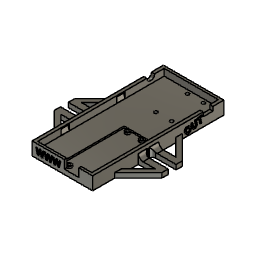
Attenuator case v8 (Autodesk Fusion 360 design; units mm, degrees)
Autodesk Fusion 360 part; units mm, degrees
note: some values were not read from the file. Set by a fixed rule: which sketch regions a step uses.
ref_plane "WorkPlane1" through (0, -11.43, -8.12) normal (0, 0, -1) x (0, -1, 0)
ref_plane "WorkPlane2" through (-25.8395, 48.6908, -2.3241) normal (-1, 0, 0) x (0, 0, 1)
ref_plane "WorkPlane3" through (-2.2175, 54.0502, -2.1844) normal (1, 0, 0) x (0, 1, 0)
sketch "Sketch2" plane through (-25.8395, 48.6908, -2.3241) normal (-1, 0, 0) x (0, 1, 0)
  line L0 (-7.62, -7.62) -> (10.16, -7.62)
  constraint horizontal L0
sketch "Sketch1" plane through (0, -11.43, -8.12) normal (0, 0, -1) x (1, 0, 0)
  line L0 (21.4045, -77.7992) -> (-25.8395, -77.7992)
  line L1 (-25.8395, -77.7992) -> (-25.8395, 28.04)
  line L2 (-25.8395, 28.04) -> (21.4045, 28.04)
  line L3 (21.4045, 28.04) -> (21.4045, -77.7992)
  line L4 (21.4045, -62.1782) -> (21.4045, -68.7822)
  line L5 (-25.8395, -52.5008) -> (-25.8395, -70.2808)
  line L6 (-0.4395, -75.2592) -> (-3.9955, -75.2592)
  line L7 (-10.5, 25.5) -> (10.5, 25.5)
  line L8 (-25.8395, -77.7992) -> (-26.6015, -77.7992)
  line L9 (-26.6015, -77.7992) -> (-26.6015, 28.04)
  line L10 (-26.6015, 28.04) -> (-25.8395, 28.04)
  line L11 (-25.8395, 28.04) -> (-25.8395, -77.7992)
  line L12 (21.4045, -77.7992) -> (22.1665, -77.7992)
  line L13 (22.1665, -77.7992) -> (22.1665, 28.04)
  line L14 (22.1665, 28.04) -> (21.4045, 28.04)
  line L15 (21.4045, 28.04) -> (21.4045, -77.7992)
  dimension "d10" = 2.54
  dimension "d11" = 2.54
  dimension "d12" = 0.762
  dimension "d13" = 0.762
  constraint horizontal L0
  constraint vertical L1
  constraint horizontal L2
  constraint vertical L3
  constraint collinear L3 L4
  constraint collinear L1 L5
  constraint horizontal L8
  constraint vertical L9
  constraint horizontal L10
  constraint vertical L11
  constraint collinear L2 L10
  constraint horizontal L12
  constraint vertical L13
  constraint horizontal L14
  constraint vertical L15
  constraint collinear L2 L14
  measures "d10" distance of L0 L6
  measures "d11" distance of L2 L7
  measures "d12" distance of L0.end L8.end
  measures "d13" distance of L0.start L12.end
extrude "Extrude2" add sketch "Sketch1" along normal blind 5.04
sketch "Sketch3" plane through (0, 0, -8.12) normal (0, 0, 1) x (-1, 0, 0)
  line L0 (-22.1665, -66.3692) -> (26.6015, -66.3692)
  line L1 (26.6015, -66.3692) -> (26.6015, 39.47)
  line L2 (26.6015, 39.47) -> (-22.1665, 39.47)
  line L3 (-22.1665, 39.47) -> (-22.1665, -66.3692)
  line L4 (26.6015, -66.3692) -> (-22.1665, -66.3692)
  line L5 (-22.1665, -66.3692) -> (-22.1665, 39.47)
  line L6 (-22.1665, 39.47) -> (26.6015, 39.47)
  line L7 (26.6015, 39.47) -> (26.6015, -66.3692)
  line L8 (25.3315, -64.4642) -> (-20.8965, -64.4642)
  line L9 (-20.8965, -64.4642) -> (-20.8965, 37.565)
  line L10 (-20.8965, 37.565) -> (25.3315, 37.565)
  line L11 (25.3315, 37.565) -> (25.3315, -64.4642)
  dimension "d16" = 1.905
  dimension "d17" = 1.905
  dimension "d18" = 1.27
  dimension "d19" = 1.27
  constraint horizontal L4
  constraint vertical L5
  constraint horizontal L6
  constraint vertical L7
  constraint coincident L2.end L3.start
  constraint coincident L0.end L1.start
  constraint horizontal L8
  constraint vertical L9
  constraint horizontal L10
  constraint vertical L11
  measures "d16" distance of L4 L8
  measures "d17" distance of L6 L10
  measures "d18" distance of L7 L11
  measures "d19" distance of L5 L9
extrude "Extrude3" add sketch "Sketch3" along normal blind 5.4356
sketch "Sketch4" plane through (22.1665, 0, 0) normal (1, 0, 0) x (0, 1, 0)
  line L0 (-39.47, -2.6844) -> (-39.47, -13.16)
  line L1 (-39.47, -13.16) -> (66.3692, -13.16)
  line L2 (66.3692, -13.16) -> (66.3692, -2.6844)
  line L3 (66.3692, -2.6844) -> (-39.47, -2.6844)
  circle A0 centre (53.6692, -2.6844) radius 3.175
  dimension "d22" = 6.35
  dimension "d23" = 12.7
  constraint coincident L3 A0.centre
  measures "d22" diameter of A0
  measures "d23" distance of L2 A0.centre
extrude "Extrude4" cut sketch "Sketch4" against normal up to surface (48.768 mm away) contours L3 A0 | L3 A0
sketch "Sketch5" plane through (22.1665, 0, 0) normal (1, 0, 0) x (0, 1, 0)
  arc A0 (50.4942, -2.6844) -> (56.8442, -2.6844) centre (53.6692, -2.6844) ccw
  line L0 (50.4942, -2.6844) -> (-39.47, -2.6844)
  line L1 (-39.47, -2.6844) -> (-39.47, -13.16)
  line L2 (-39.47, -13.16) -> (66.3692, -13.16)
  line L3 (66.3692, -13.16) -> (66.3692, -2.6844)
  line L4 (66.3692, -2.6844) -> (56.8442, -2.6844)
  line L5 (49.7322, -2.6844) -> (57.6062, -2.6844)
  line L6 (57.6062, -2.6844) -> (57.6062, -6.0198)
  line L7 (57.6062, -6.0198) -> (49.7322, -6.0198)
  line L8 (49.7322, -6.0198) -> (49.7322, -2.6844)
  line L9 (50.7482, 1.016) -> (57.3522, 1.016)
  line L10 (50.7482, 1.016) -> (50.7482, -5.3848)
  line L11 (57.3522, 1.016) -> (57.3522, -5.3848)
  line L12 (50.7482, -5.3848) -> (57.3522, -5.3848)
  dimension "d137" = 7.874
  dimension "d138" = 3.3354
  dimension "d139" = 8.763
  constraint horizontal L5
  constraint vertical L6
  constraint horizontal L7
  constraint vertical L8
  constraint collinear L4 L5
  measures "d137" distance of L6.end L7.end
  measures "d138" distance of L4 L7
  measures "d139" distance of L3 L6
extrude "Extrude5" cut sketch "Sketch5" against normal up to surface (1.27 mm away) contours A0 L0 L4 L5 L6 L7 L8 L10 L11 L12 | A0 L10 L12 | A0 L4 L5 L11 L12
sketch "Sketch10" plane through (0, -39.47, 0) normal (0, -1, 0) x (1, 0, 0)
  line L0 (22.1665, -2.6844) -> (-26.6015, -2.6844)
  line L1 (-26.6015, -2.6844) -> (-26.6015, -13.16)
  line L2 (-26.6015, -13.16) -> (22.1665, -13.16)
  line L3 (22.1665, -13.16) -> (22.1665, -2.6844)
  line L4 (-0.4634, -2.6844) -> (10.9837, -2.6844)
  line L5 (10.9837, -2.6844) -> (10.9837, -13.16)
  line L6 (10.9837, -13.16) -> (-0.4634, -13.16)
  line L7 (-0.4634, -13.16) -> (-0.4634, -2.6844)
  constraint horizontal L4
  constraint vertical L5
  constraint horizontal L6
  constraint vertical L7
  constraint coincident L2 L5.end
extrude "Extrude9" cut sketch "Sketch10" against normal up to surface (1.905 mm away) contours L0 L2 L4 L5 L6 L7
sketch "Sketch11" plane through (0, 0, -13.16) normal (0, 0, -1) x (1, 0, 0)
  line L0 (10.9837, 39.47) -> (10.9837, 37.565)
  line L1 (10.9837, 37.565) -> (-0.4634, 37.565)
  line L2 (-0.4634, 37.565) -> (-0.4634, 39.47)
  line L3 (-0.4634, 39.47) -> (-26.6015, 39.47)
  line L4 (-26.6015, 39.47) -> (-26.6015, -66.3692)
  line L5 (-26.6015, -66.3692) -> (22.1665, -66.3692)
  line L6 (22.1665, -66.3692) -> (22.1665, 39.47)
  line L7 (22.1665, 39.47) -> (10.9837, 39.47)
  line L8 (-26.6015, 2.64) -> (-45.6515, 2.64)
  line L9 (-45.6515, 2.64) -> (-45.6515, -13.87)
  line L10 (-45.6515, -13.87) -> (-26.6015, -13.87)
  line L11 (-26.6015, -13.87) -> (-26.6015, 2.64)
  line L12 (-45.6515, -8.79) -> (-26.6015, -8.79)
  line L13 (-26.6015, -8.79) -> (-26.6015, -2.44)
  line L14 (-26.6015, -2.44) -> (-45.6515, -2.44)
  line L15 (-45.6515, -2.44) -> (-45.6515, -8.79)
  line L16 (22.1665, 2.64) -> (41.2165, 2.64)
  line L17 (41.2165, 2.64) -> (41.2165, -13.87)
  line L18 (41.2165, -13.87) -> (22.1665, -13.87)
  line L19 (22.1665, -13.87) -> (22.1665, 2.64)
  line L20 (22.1665, -2.44) -> (41.2165, -2.44)
  line L21 (41.2165, -2.44) -> (41.2165, -8.79)
  line L22 (41.2165, -8.79) -> (22.1665, -8.79)
  line L23 (22.1665, -8.79) -> (22.1665, -2.44)
  line L24 (-45.6515, 2.64) -> (-26.6015, 21.69)
  line L25 (-45.6515, 2.64) -> (-18.7108, 2.64) construction
  line L26 (-40.2634, 2.64) -> (-26.6015, 16.3018)
  line L27 (-45.6515, -13.87) -> (-26.6015, -32.92)
  line L28 (-45.6515, -13.87) -> (-18.7108, -13.87) construction
  line L29 (-40.2634, -13.87) -> (-26.6015, -27.5318)
  line L30 (41.2165, -13.87) -> (22.1665, -32.92)
  line L31 (41.2165, -13.87) -> (68.1572, -13.87) construction
  line L32 (35.8283, -13.87) -> (22.1665, -27.5318)
  line L33 (41.2165, 2.64) -> (22.1665, 21.69)
  line L34 (35.8283, 2.64) -> (22.1665, 16.3018)
  dimension "d46" = 16.51
  dimension "d47" = 6.35
  dimension "d48" = 36.83
  dimension "d49" = 19.05
  dimension "d107" = 45
  dimension "d108" = 3.81
  dimension "d109" = 45
  dimension "d110" = 3.81
  dimension "d111" = 135
  constraint horizontal L8
  constraint vertical L9
  constraint horizontal L10
  constraint vertical L11
  constraint coincident L4 L8.start
  constraint horizontal L12
  constraint vertical L13
  constraint horizontal L14
  constraint vertical L15
  constraint coincident L4 L13.end
  constraint coincident L9 L12.start
  constraint horizontal L16
  constraint vertical L17
  constraint horizontal L18
  constraint vertical L19
  constraint coincident L6 L16.start
  constraint horizontal L20
  constraint vertical L21
  constraint horizontal L22
  constraint vertical L23
  constraint coincident L17 L21.end
  constraint coincident L6 L20.start
  constraint collinear L8 L16
  constraint collinear L10 L18
  constraint collinear L12 L22
  constraint collinear L14 L20
  constraint midpoint L11 L13
  constraint equal L8 L16
  constraint horizontal L25
  constraint coincident L4 L24.end
  constraint coincident L25 L26.start
  constraint coincident L4 L26.end
  constraint parallel L24 L26
  constraint horizontal L28
  constraint coincident L4 L27.end
  constraint coincident L28 L29.start
  constraint coincident L4 L29.end
  constraint parallel L27 L29
  constraint horizontal L31
  constraint coincident L6 L30.end
  constraint coincident L18 L32.start
  constraint coincident L6 L32.end
  constraint parallel L30 L32
  constraint coincident L6 L33.end
  constraint perpendicular L32 L33
  constraint coincident L16 L34.start
  constraint coincident L6 L34.end
  constraint parallel L33 L34
  constraint equal L26 L34
  constraint equal L29 L32
  measures "d46" distance of L8.end L9.end
  measures "d47" distance of L12.start L14.end
  measures "d48" distance of L3.end L8.start
  measures "d49" distance of L8.start L8.end
  measures "d107" angle of L24 L25
  measures "d108" distance of L24 L26
  measures "d109" angle of L27 L28
  measures "d110" distance of L27 L29
  measures "d111" angle of L30 L31
extrude "Extrude10" add sketch "Sketch11" against normal blind 3.81 contours L6 L16 L33 L34 | L6 L16 L17 L19 L20 | L4 L8 L24 L26 | L6 L17 L18 L19 L22 | L4 L8 L9 L11 L14 | L6 L18 L30 L32 | L4 L9 L10 L11 L12 | L4 L10 L27 L29
fillet "Fillet1" radius 3.81 4 edges at (22.1665, -0.1, -9.35) (22.1665, 11.33, -9.35) (-26.6015, 11.33, -9.35) (-26.6015, -0.1, -9.35)
fillet "Fillet2" radius 2.54 4 edges at (-26.6015, 2.44, -9.35) (-26.6015, 8.79, -9.35) (22.1665, 2.44, -9.35) (22.1665, 8.79, -9.35)
sketch "Sketch13" plane through (0, 0, -8.12) normal (0, 0, 1) x (-1, 0, 0)
  line L0 (-20.8965, 37.565) -> (-20.8965, -64.4642)
  line L1 (-20.8965, -64.4642) -> (25.3315, -64.4642)
  line L2 (25.3315, -64.4642) -> (25.3315, 37.565)
  line L3 (25.3315, 37.565) -> (0.4634, 37.565)
  line L4 (0.4634, 37.565) -> (-10.9837, 37.565)
  line L5 (-10.9837, 37.565) -> (-20.8965, 37.565)
  circle A0 centre (-10.8539, 35.565) radius 1.05
  circle A1 centre (0.5461, 35.565) radius 1.05
  circle A2 centre (0.5461, -11.435) radius 1.05
  circle A3 centre (-10.4825, -61.5432) radius 1.3462
  circle A4 centre (2.2175, -36.0416) radius 1.3462
  circle A5 centre (-10.4825, -36.0416) radius 1.3462
  circle A6 centre (-10.8539, -11.435) radius 1.05
  circle A7 centre (2.2175, -61.5432) radius 1.3462
  circle A8 centre (-10.8539, 35.565) radius 1.05
  circle A9 centre (0.5461, 35.565) radius 1.05
  circle A10 centre (0.5461, -11.435) radius 1.05
  circle A11 centre (-10.8539, -11.435) radius 1.05
  circle A12 centre (-10.4825, -36.0416) radius 1.3462
  circle A13 centre (2.2175, -36.0416) radius 1.3462
  circle A14 centre (2.2175, -61.5432) radius 1.3462
  circle A15 centre (-10.4825, -61.5432) radius 1.3462
  constraint concentric A0 A8
  constraint concentric A1 A9
  constraint concentric A2 A10
  constraint concentric A6 A11
  constraint concentric A5 A12
  constraint concentric A4 A13
  constraint concentric A7 A14
  constraint concentric A3 A15
  constraint equal A7 A14
  constraint equal A3 A15
  constraint equal A5 A12
  constraint equal A4 A13
  constraint equal A2 A10
  constraint equal A6 A11
  constraint equal A1 A9
  constraint equal A0 A8
extrude "Extrude12" cut sketch "Sketch13" against normal up to surface (5.04 mm away) contours A0 A8 | A1 A9 | A2 A10 | A3 A15 | A4 A13 | A5 A12 | A6 A11 | A7 A14
sketch "Sketch14" plane through (0, 0, -13.16) normal (0, 0, -1) x (1, 0, 0)
  line L0 (-0.4634, 39.47) -> (-26.6015, 39.47)
  line L1 (-26.6015, 39.47) -> (-26.6015, 21.69)
  line L2 (-26.6015, 2.64) -> (-40.2634, 2.64)
  line L3 (-45.6515, 2.64) -> (-45.6515, -2.44)
  line L4 (-45.6515, -2.44) -> (-29.1415, -2.44)
  arc A0 (-26.6015, -4.98) -> (-29.1415, -2.44) centre (-29.1415, -4.98) ccw
  line L5 (-26.6015, -4.98) -> (-26.6015, -6.25)
  arc A1 (-29.1415, -8.79) -> (-26.6015, -6.25) centre (-29.1415, -6.25) ccw
  line L6 (-29.1415, -8.79) -> (-45.6515, -8.79)
  line L7 (-45.6515, -8.79) -> (-45.6515, -13.87)
  line L8 (-40.2634, -13.87) -> (-26.6015, -13.87)
  line L9 (-26.6015, -13.87) -> (-26.6015, -27.5318)
  line L10 (22.1665, 21.69) -> (22.1665, 39.47)
  line L11 (22.1665, -13.87) -> (35.8283, -13.87)
  line L12 (41.2165, -13.87) -> (41.2165, -8.79)
  line L13 (41.2165, -8.79) -> (24.7065, -8.79)
  arc A2 (22.1665, -6.25) -> (24.7065, -8.79) centre (24.7065, -6.25) ccw
  line L14 (22.1665, -6.25) -> (22.1665, -4.98)
  arc A3 (24.7065, -2.44) -> (22.1665, -4.98) centre (24.7065, -4.98) ccw
  line L15 (24.7065, -2.44) -> (41.2165, -2.44)
  line L16 (41.2165, -2.44) -> (41.2165, 2.64)
  line L17 (35.8283, 2.64) -> (22.1665, 2.64)
  line L18 (22.1665, 2.64) -> (22.1665, 16.3018)
  line L19 (22.1665, 39.47) -> (10.9837, 39.47)
  line L20 (9.0102, -58.9932) -> (7.538, -61.5432)
  line L21 (7.538, -61.5432) -> (9.0102, -64.0932)
  line L22 (9.0102, -64.0932) -> (11.9547, -64.0932)
  line L23 (11.9547, -64.0932) -> (13.427, -61.5432)
  line L24 (13.427, -61.5432) -> (11.9547, -58.9932)
  line L25 (11.9547, -58.9932) -> (9.0102, -58.9932)
  line L26 (9.0102, -38.5916) -> (11.9547, -38.5916)
  line L27 (9.0102, -33.4916) -> (7.538, -36.0416)
  line L28 (13.427, -36.0416) -> (11.9547, -33.4916)
  line L29 (11.9547, -38.5916) -> (13.427, -36.0416)
  line L30 (7.538, -36.0416) -> (9.0102, -38.5916)
  line L31 (11.9547, -33.4916) -> (9.0102, -33.4916)
  line L32 (0.727, -61.5432) -> (-0.7453, -58.9932)
  line L33 (-3.6898, -64.0932) -> (-0.7453, -64.0932)
  line L34 (-3.6898, -58.9932) -> (-5.162, -61.5432)
  line L35 (-0.7453, -58.9932) -> (-3.6898, -58.9932)
  line L36 (-0.7453, -64.0932) -> (0.727, -61.5432)
  line L37 (-5.162, -61.5432) -> (-3.6898, -64.0932)
  line L38 (-3.6898, -38.5916) -> (-0.7453, -38.5916)
  line L39 (-3.6898, -33.4916) -> (-5.162, -36.0416)
  line L40 (0.727, -36.0416) -> (-0.7453, -33.4916)
  line L41 (-0.7453, -38.5916) -> (0.727, -36.0416)
  line L42 (-5.162, -36.0416) -> (-3.6898, -38.5916)
  line L43 (-0.7453, -33.4916) -> (-3.6898, -33.4916)
  circle A4 centre (-2.2175, -61.5432) radius 2.55
  circle A5 centre (-2.2175, -61.5432) radius 1.3462
  line L44 (-26.6015, -66.3692) -> (22.1665, -66.3692)
  circle A6 centre (10.4825, -36.0416) radius 2.55
  circle A7 centre (10.4825, -36.0416) radius 1.3462
  line L45 (0.6374, 33.515) -> (1.821, 35.565)
  line L46 (1.821, 35.565) -> (0.6374, 37.615)
  line L47 (0.6374, 37.615) -> (-1.7297, 37.615)
  line L48 (-1.7297, 37.615) -> (-2.9133, 35.565)
  line L49 (-2.9133, 35.565) -> (-1.7297, 33.515)
  line L50 (-1.7297, 33.515) -> (0.6374, 33.515)
  circle A8 centre (-0.5461, 35.565) radius 2.05
  line L51 (8.4867, -11.435) -> (9.6703, -13.485)
  circle A9 centre (10.8539, -11.435) radius 2.05
  line L52 (13.221, -11.435) -> (12.0374, -9.385)
  line L53 (9.6703, -13.485) -> (12.0374, -13.485)
  line L54 (12.0374, -9.385) -> (9.6703, -9.385)
  line L55 (12.0374, -13.485) -> (13.221, -11.435)
  line L56 (9.6703, -9.385) -> (8.4867, -11.435)
  line L57 (13.221, 35.565) -> (12.0374, 37.615)
  line L58 (12.0374, 37.615) -> (9.6703, 37.615)
  line L59 (9.6703, 37.615) -> (8.4867, 35.565)
  line L60 (8.4867, 35.565) -> (9.6703, 33.515)
  line L61 (9.6703, 33.515) -> (12.0374, 33.515)
  line L62 (12.0374, 33.515) -> (13.221, 35.565)
  line L63 (1.821, -11.435) -> (0.6374, -9.385)
  line L64 (0.6374, -9.385) -> (-1.7297, -9.385)
  line L65 (-1.7297, -9.385) -> (-2.9133, -11.435)
  line L66 (-2.9133, -11.435) -> (-1.7297, -13.485)
  line L67 (-1.7297, -13.485) -> (0.6374, -13.485)
  line L68 (0.6374, -13.485) -> (1.821, -11.435)
  circle A10 centre (-0.5461, 35.565) radius 1.05
  circle A11 centre (10.8539, -11.435) radius 1.05
  line L69 (-26.6015, 21.69) -> (-45.6515, 2.64)
  line L70 (-45.6515, -13.87) -> (-26.6015, -32.92)
  line L71 (-26.6015, -32.92) -> (-26.6015, -66.3692)
  line L72 (22.1665, -66.3692) -> (22.1665, -32.92)
  line L73 (22.1665, -32.92) -> (41.2165, -13.87)
  line L74 (41.2165, 2.64) -> (22.1665, 21.69)
  line L75 (22.1665, 16.3018) -> (35.8283, 2.64)
  line L76 (22.1665, -27.5318) -> (22.1665, -13.87)
  line L77 (35.8283, -13.87) -> (22.1665, -27.5318)
  line L78 (-26.6015, 16.3018) -> (-26.6015, 2.64)
  line L79 (-40.2634, 2.64) -> (-26.6015, 16.3018)
  line L80 (-26.6015, -27.5318) -> (-40.2634, -13.87)
  point P0 (10.4825, -61.5432)
  point P1 (10.4825, -36.0416)
  point P2 (-2.2175, -61.5432)
  point P3 (-2.2175, -36.0416)
  point P4 (-0.5461, 35.565)
  point P5 (10.8539, -11.435)
  point P6 (10.8539, 35.565)
  point P7 (-0.5461, -11.435)
  dimension "d91" = 2.55
  dimension "d92" = 2.55
  dimension "d93" = 2.55
  dimension "d94" = 2.55
  dimension "d99" = 2.05
  dimension "d100" = 2.05
  dimension "d101" = 2.05
  dimension "d102" = 2.05
  constraint coincident P2 A4.centre
  constraint tangent L37 A4
  constraint concentric A4 A5
  constraint parallel L33 L44
  constraint horizontal P0 P2
  constraint vertical P2 P3
  constraint horizontal P1 P3
  constraint vertical P0 P1
  constraint parallel L25 L33
  constraint parallel L25 L31
  constraint parallel L35 L43
  constraint coincident P1 A6.centre
  constraint tangent L31 A6
  constraint concentric A6 A7
  constraint coincident P4 A8.centre
  constraint tangent L50 A8
  constraint coincident P5 A9.centre
  constraint tangent A9 L55
  constraint horizontal P4 P6
  constraint vertical P5 P6
  constraint horizontal P5 P7
  constraint vertical P4 P7
  constraint parallel L0 L50
  constraint parallel L19 L58
  constraint parallel L54 L61
  constraint parallel L50 L64
  constraint concentric A8 A10
  constraint concentric A9 A11
  measures "d91" distance of P0 L25
  measures "d92" distance of P1 L31
  measures "d93" distance of P2 L37
  measures "d94" distance of P3 L43
  measures "d99" distance of P4 L50
  measures "d100" distance of P5 L55
  measures "d101" distance of P6 L62
  measures "d102" distance of P7 L68
extrude "Extrude13" cut sketch "Sketch14" against normal blind 3 contours L20 L21 L22 L23 L24 L25 | L26 L30 A6 | L26 L29 A6 | A6 | L27 L30 A6 | L28 L29 A6 | L27 L31 A6 | L28 L31 A6 | L32 L36 A4 | L32 L35 A4 | A4 | L33 L36 A4 | L34 L35 A4 | L33 L37 A4 | L34 L37 A4 | L38 L39 L40 L41 L42 L43 | A5 | A7
sketch "Sketch15" plane through (0, -39.47, 0) normal (0, -1, 0) x (1, 0, 0)
  line L0 (10.9837, -2.6844) -> (10.9837, -13.16)
  line L1 (10.9837, -13.16) -> (22.1665, -13.16)
  line L2 (22.1665, -13.16) -> (22.1665, -2.6844)
  line L3 (22.1665, -2.6844) -> (10.9837, -2.6844)
  line L4 (-26.6015, -13.16) -> (-0.4634, -13.16) construction
  line L5 (-0.4634, -13.16) -> (-0.4634, -2.6844) construction
  line L6 (-0.4634, -2.6844) -> (-26.6015, -2.6844) construction
  line L7 (-26.6015, -2.6844) -> (-26.6015, -13.16) construction
  point P0 (-0.4634, -13.16)
  point P1 (-26.6015, -2.6844)
  point P2 (-0.4634, -2.6844)
  dimension "d68" = 5.08
  text T0 "WWW" font "Arial" height 5.08 bold align centre middle in box 26.1382 x 10.4756 at (-26.6015, -13.16) x (1, 0) y (0, 1) spacing 1
  constraint coincident L4 P0
  constraint coincident P0
  constraint coincident P1
  constraint coincident P2
extrude "Extrude14" cut sketch "Sketch15" against normal blind 1.016 text T0
sketch "Sketch16" plane through (22.1665, 0, 0) normal (1, 0, 0) x (0, 1, 0)
  line L0 (6.25, -13.16) -> (6.25, -5.54)
  line L1 (6.25, -5.54) -> (13.87, -5.54)
  line L2 (13.87, -5.54) -> (13.87, -13.16)
  line L3 (13.87, -13.16) -> (27.5318, -13.16)
  line L4 (66.3692, -13.16) -> (66.3692, -2.6844)
  line L5 (66.3692, -2.6844) -> (57.6062, -2.6844)
  line L6 (57.6062, -2.6844) -> (57.6062, -6.0198)
  line L7 (57.6062, -6.0198) -> (49.7322, -6.0198)
  line L8 (49.7322, -6.0198) -> (49.7322, -2.6844)
  line L9 (49.7322, -2.6844) -> (-39.47, -2.6844)
  line L10 (-39.47, -2.6844) -> (-39.47, -13.16)
  line L11 (-16.3018, -13.16) -> (-2.64, -13.16)
  line L12 (-2.64, -13.16) -> (-2.64, -5.54)
  line L13 (-2.64, -5.54) -> (4.98, -5.54)
  line L14 (4.98, -5.54) -> (4.98, -13.16)
  line L15 (4.98, -13.16) -> (6.25, -13.16)
  line L16 (36.1717, -13.16) -> (49.0012, -10.4931) construction
  line L17 (49.0012, -10.4931) -> (47.378, -2.6844) construction
  line L18 (47.378, -2.6844) -> (34.5485, -5.3513) construction
  line L19 (34.5485, -5.3513) -> (36.1717, -13.16) construction
  line L20 (27.5318, -13.16) -> (27.5318, -9.35)
  line L21 (27.5318, -9.35) -> (32.92, -9.35)
  line L22 (32.92, -9.35) -> (32.92, -13.16)
  line L23 (32.92, -13.16) -> (66.3692, -13.16)
  line L24 (-39.47, -13.16) -> (-21.69, -13.16)
  line L25 (-21.69, -13.16) -> (-21.69, -9.35)
  line L26 (-21.69, -9.35) -> (-16.3018, -9.35)
  line L27 (-16.3018, -9.35) -> (-16.3018, -13.16)
  dimension "d71" = 5.08
  text T0 "OUT" font "Arial" height 5.08 bold align centre middle in box 13.1037 x 7.9756 at (36.1717, -13.16) x (0.97907, 0.203524) y (-0.203524, 0.97907) spacing 1
  constraint coincident L9
  constraint coincident L3
extrude "Extrude15" add sketch "Sketch16" along normal blind 0.508 text T0
sketch "Sketch17" plane through (-26.6015, 0, 0) normal (-1, 0, 0) x (0, -1, 0)
  line L0 (-6.25, -5.54) -> (-6.25, -13.16)
  line L1 (-6.25, -13.16) -> (-4.98, -13.16)
  line L2 (-4.98, -13.16) -> (-4.98, -5.54)
  line L3 (-4.98, -5.54) -> (2.64, -5.54)
  line L4 (2.64, -5.54) -> (2.64, -13.16)
  line L5 (21.69, -13.16) -> (39.47, -13.16)
  line L6 (39.47, -13.16) -> (39.47, -2.6844)
  line L7 (39.47, -2.6844) -> (-50.4942, -2.6844)
  arc A0 (-56.8442, -2.6844) -> (-50.4942, -2.6844) centre (-53.6692, -2.6844) ccw
  line L8 (-56.8442, -2.6844) -> (-66.3692, -2.6844)
  line L9 (-66.3692, -2.6844) -> (-66.3692, -13.16)
  line L10 (-27.5318, -13.16) -> (-13.87, -13.16)
  line L11 (-13.87, -13.16) -> (-13.87, -5.54)
  line L12 (-13.87, -5.54) -> (-6.25, -5.54)
  line L13 (-50.628, -10.3581) -> (-40.7366, -13.16) construction
  line L14 (-40.7366, -13.16) -> (-38.5629, -5.4863) construction
  line L15 (-38.5629, -5.4863) -> (-48.4542, -2.6844) construction
  line L16 (-48.4542, -2.6844) -> (-50.628, -10.3581) construction
  line L17 (2.64, -13.16) -> (16.3018, -13.16)
  line L18 (16.3018, -13.16) -> (16.3018, -9.35)
  line L19 (16.3018, -9.35) -> (21.69, -9.35)
  line L20 (21.69, -9.35) -> (21.69, -13.16)
  line L21 (-66.3692, -13.16) -> (-32.92, -13.16)
  line L22 (-32.92, -13.16) -> (-32.92, -9.35)
  line L23 (-32.92, -9.35) -> (-27.5318, -9.35)
  line L24 (-27.5318, -9.35) -> (-27.5318, -13.16)
  dimension "d74" = 5.08
  text T0 "IN" font "Arial" height 5.08 bold align centre middle in box 10.2805 x 7.9756 at (-50.628, -10.3581) x (0.962142, -0.272549) y (0.272549, 0.962142) spacing 1
  constraint coincident L10
  constraint coincident L7
extrude "Extrude16" add sketch "Sketch17" along normal blind 0.508 text T0
extrude "Extrude17" cut sketch "Sketch14" against normal blind 3 contours L45 L50 A8 | L45 L46 A8 | A8 | L49 L50 A8 | L48 L49 A8 | L46 L47 A8 | L47 L48 A8 | L51 A9 L56 | L51 A9 L53 | A9 | A9 L54 L56 | A9 L53 L55 | A9 L52 L54 | A9 L52 L55 | L57 L58 L59 L60 L61 L62 | L63 L64 L65 L66 L67 L68 | A10 | A11
sketch "Sketch18" plane through (0, 0, -8.12) normal (0, 0, 1) x (-1, 0, 0)
  circle A0 centre (-10.8539, 35.565) radius 1.05
  circle A1 centre (-10.4825, -61.5432) radius 1.3462
  circle A2 centre (2.2175, -36.0416) radius 1.3462
  circle A3 centre (-10.8539, -11.435) radius 1.05
  circle A4 centre (0.5461, 35.565) radius 1.05
  circle A5 centre (2.2175, -61.5432) radius 1.3462
  circle A6 centre (-10.4825, -36.0416) radius 1.3462
  circle A7 centre (0.5461, -11.435) radius 1.05
  line L0 (-20.8965, 37.565) -> (-20.8965, -64.4642)
  line L1 (-20.8965, -64.4642) -> (25.3315, -64.4642)
  line L2 (25.3315, -64.4642) -> (25.3315, 37.565)
  line L3 (25.3315, 37.565) -> (0.4634, 37.565)
  line L4 (0.4634, 37.565) -> (-10.9837, 37.565)
  line L5 (-10.9837, 37.565) -> (-20.8965, 37.565)
  circle A8 centre (0.5461, -11.435) radius 2
  circle A9 centre (-10.8539, -11.435) radius 2
  circle A10 centre (-10.8539, 35.565) radius 2
  circle A11 centre (0.5461, 35.565) radius 2
  line L6 (5.3461, -13.435) -> (-15.6539, -13.435)
  line L7 (-15.6539, -13.435) -> (-15.6539, 37.565)
  line L8 (-15.6539, 37.565) -> (5.3461, 37.565)
  line L9 (5.3461, 37.565) -> (5.3461, -13.435)
  line L10 (5.3461, 35.565) -> (2.5461, 35.565)
  line L11 (2.5461, 32.9801) -> (2.5461, 37.565)
  line L12 (-12.8539, 33.02) -> (-12.8539, 37.565)
  line L13 (-15.6539, 35.565) -> (-12.8539, 35.565)
  dimension "d112" = 21
  dimension "d113" = 51
  constraint concentric A7 A8
  constraint concentric A3 A9
  constraint concentric A0 A10
  constraint concentric A4 A11
  constraint horizontal L6
  constraint vertical L7
  constraint horizontal L8
  constraint vertical L9
  constraint tangent A8 L6
  constraint tangent A9 L6
  constraint tangent A10 L8
  constraint tangent A11 L8
  constraint collinear L3 L8
  constraint coincident L9 L10.start
  constraint coincident A11 L10.end
  constraint perpendicular L9 L10
  constraint coincident L8 L11.end
  constraint coincident L3 L11.end
  constraint tangent A11 L11
  constraint perpendicular L10 L11
  constraint coincident L5 L12.end
  constraint coincident L7 L13.start
  constraint coincident L12 L13.end
  constraint perpendicular L12 L13
  constraint perpendicular L7 L13
  constraint tangent A10 L12
  constraint equal L10 L13
  constraint coincident L10.end L11
  constraint coincident A10 L13.end
  measures "d112" distance of L6.start L6.end
  measures "d113" distance of L6.start L8.end
extrude "Extrude18" cut sketch "Sketch18" against normal blind 1.27 contours L3 A11 L8 L11 | L5 L7 L8 L12 L13 | L4 L5 A10 L8 L12 | L4 A10 A11 L6 L7 L8 L9 L10 L13 | L3 L8 L9 L10 L11
sketch "Sketch19" plane through (0, -37.565, 0) normal (0, -1, 0) x (1, 0, 0)
  line L0 (10.8539, -9.39) -> (-0.4634, -9.39)
  line L1 (-0.4634, -9.39) -> (-0.4634, -10.16)
  line L2 (-0.4634, -10.16) -> (0.6663, -10.16)
  line L3 (0.6663, -10.16) -> (0.6663, -13.16)
  line L4 (0.6663, -13.16) -> (9.6414, -13.16)
  line L5 (9.6414, -13.16) -> (9.6414, -10.16)
  line L6 (9.6414, -10.16) -> (10.9837, -10.16)
  line L7 (10.9837, -10.16) -> (10.9837, -9.39)
  line L8 (10.9837, -9.39) -> (10.8539, -9.39)
  line L9 (-0.4634, -9.39) -> (10.9837, -9.39)
  line L10 (10.9837, -9.39) -> (10.9837, -13.16)
  line L11 (10.9837, -13.16) -> (-0.4634, -13.16)
  line L12 (-0.4634, -13.16) -> (-0.4634, -9.39)
  point P0 (10.9837, -13.16)
  constraint horizontal L9
  constraint vertical L10
  constraint horizontal L11
  constraint vertical L12
  constraint coincident L0.end L1.start
  constraint coincident P0 L10.end
extrude "Extrude19" add sketch "Sketch19" along normal up to surface (1.905 mm away)
extrude "Extrude20" cut sketch "Sketch14" against normal up to surface (3 mm away) contours A8 | L46 L47 A8 | L47 L48 A8 | L57 L58 L59 L60 L61 L62
extrude "Extrude21" add 1 faces at (-25.3315, -8.2119, -4.4963) along direction (1, 0, 0) blind 1.27
extrude "Extrude22" add 1 faces at (20.8965, -8.4659, -5.6081) along direction (-1, 0, 0) blind 1.27
ref_plane "WorkPlane4" through (-12.8974, -15.34, -6.0372) normal (0, 1, 0) x (-1, 0, 0)
sketch "Sketch20" plane through (-12.8974, -15.34, -6.0372) normal (0, 1, 0) x (1, 0, 0)
  line L0 (32.5239, -3.3528) -> (33.5653, -1.4351)
  line L1 (33.5653, -1.4351) -> (32.5239, 1.9812)
  line L2 (32.5239, 1.9812) -> (32.5239, -3.3528)
  line L3 (-11.1641, -3.3528) -> (-11.1641, 1.9812)
  line L4 (-11.1641, 1.9812) -> (-12.2055, -1.4351)
  line L5 (-12.2055, -1.4351) -> (-11.1641, -3.3528)
  line L6 (32.5239, 2.0828) -> (32.5239, -3.3528)
  line L7 (-11.1641, -3.3528) -> (-11.1641, 2.0828)
  dimension "d126" = 1.0414
  dimension "d127" = 5.334
  dimension "d128" = 1.9177
  constraint vertical L2
  constraint vertical L3
  constraint equal L2 L3
  constraint equal L1 L4
  constraint equal L0 L5
  constraint horizontal L0.start L3.start
  constraint collinear L2 L6
  constraint collinear L3 L7
  constraint coincident L3.start L5.end
  measures "d126" distance of L0.end L2
  measures "d127" distance of L0.start L1.end
  measures "d128" vertical distance of L0.start L0.end
extrude "Extrude23" cut sketch "Sketch20" along normal mid plane 6.604
ref_plane "WorkPlane5" through (-2.2175, 29.5392, -5.4022) normal (0, -1, 0) x (1, 0, 0)
sketch "Sketch21" plane through (-2.2175, 29.5392, -5.4022) normal (0, -1, 0) x (-1, 0, 0)
  line L0 (21.844, -2.7178) -> (21.844, 2.6162)
  line L1 (21.844, 2.6162) -> (22.8854, -0.8001)
  line L2 (22.8854, -0.8001) -> (21.844, -2.7178)
  line L3 (-21.844, -2.7178) -> (-21.844, 2.6162)
  line L4 (-21.844, 2.6162) -> (-22.8854, -0.8001)
  line L5 (-22.8854, -0.8001) -> (-21.844, -2.7178)
  line L6 (-21.844, -2.7178) -> (-21.844, 2.7178)
  line L7 (21.844, 2.7178) -> (21.844, -2.7178)
  dimension "d132" = 5.334
  dimension "d133" = 1.0414
  dimension "d134" = 1.9177
  constraint vertical L0
  constraint parallel L0 L3
  constraint equal L0 L3
  constraint horizontal L0.start L3.start
  constraint equal L2 L5
  constraint equal L1 L4
  constraint collinear L3 L6
  constraint collinear L0 L7
  constraint coincident L3.start L5.end
  constraint coincident L1.end L2.start
  measures "d132" distance of L3.start L3.end
  measures "d133" distance of L3 L4.end
  measures "d134" vertical distance of L3.start L4.end
extrude "Extrude24" cut sketch "Sketch21" along normal mid plane 6.604
equation "d14 = 0.1 in + 2.5 mm"
equation "d125 = ( 7 / 8 ) * 1 in"
equation "d129 = ( 0.26 / 2 ) * 1 in"
equation "d131 = ( 11 / 8 ) * 1 in"
equation "d135 = ( 0.26 / 2 ) * 1 in"
